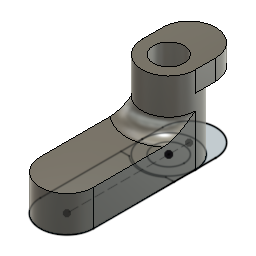
OBS-Mounting-A-003_LockingPin_v0.1.0 (Autodesk Fusion 360 design; units mm, degrees)
Autodesk Fusion 360 part; units mm, degrees
sketch "Skizze1" plane through (0, 0, 0) normal (0, 1, 0) x (1, 0, 0)
  circle A0 centre (0, 0) radius 1.5
  line L0 (2.6, 0) -> (2.6, 2)
  arc A1 (2.6, 2) -> (-2.6, 2) centre (0, 2) ccw
  line L1 (-2.6, 2) -> (-2.6, 0)
  arc A2 (-2.6, 0) -> (2.6, 0) centre (0, 0) ccw
  line L2 (0, 0) -> (0, 2) construction
  line L3 (-2.6, 0) -> (-2.6, -10)
  arc A3 (-2.6, -10) -> (2.6, -10) centre (0, -10) ccw
  line L4 (2.6, -10) -> (2.6, 0)
  arc A4 (2.6, 0) -> (-2.6, 0) centre (0, 0) ccw
  line L5 (0, 0) -> (0, -10) construction
  line L6 (-2.6, -2.0791) -> (-1.8, -2.0791)
  line L7 (2.6, -2.0791) -> (2.4645, -2.0791)
  line L8 (2.4645, -2.0791) -> (1.8, -2.0791)
  arc A5 (-1.8, -2.0791) -> (1.8, -2.0791) centre (0, 0) ccw
  dimension "d1" = 3
  dimension "d2" = 2
  dimension "d3" = 10
  dimension "d4" = 2.6
  dimension "d13" = 2.75
  dimension "d14" = 0.8
  constraint coincident A0.centre A2.centre
  constraint tangent L0 A1
  constraint tangent A1 L1
  constraint parallel L0 L1
  constraint tangent L1 A2
  constraint tangent L0 A2
  constraint vertical L2
  constraint tangent L3 A3
  constraint tangent A3 L4
  constraint parallel L3 L4
  constraint tangent L4 A4
  constraint tangent L3 A4
  constraint parallel L2 L5
  constraint equal A2 A4
  constraint coincident L3 L6.start
  constraint perpendicular L3 L6
  constraint coincident L4 L7.start
  constraint perpendicular L4 L7
  constraint perpendicular L4 L8
  constraint concentric A0 A5
  constraint collinear L6 L8
  measures "d1" diameter of A0
  measures "d2" distance of A0.centre A1.centre
  measures "d3" distance of A0.centre A3.centre
  measures "d4" radius of A1
  measures "d13" radius of A5
  measures "d14" distance of L6.start L6.end
extrude "Extrusion1" add sketch "Skizze1" along normal blind 3.5 contours A2 L3 L4 L6 L7 L8 A5 | A2 A4 | L3 A3 L4 L6 L7 L8 A5
extrude "Extrusion2" add sketch "Skizze1" along normal blind 6.5 contours A2 A4
extrude "Extrusion3" add sketch "Skizze1" along normal blind 2 from surface at 6.5 contours L0 A1 L1 A4 | A2 A4
fillet "Abrundung1" radius 1.5 1 edges at (0, 3.5, 2.6)
equation "d13 = ( 5.5 / 2 ) * 1 mm"
